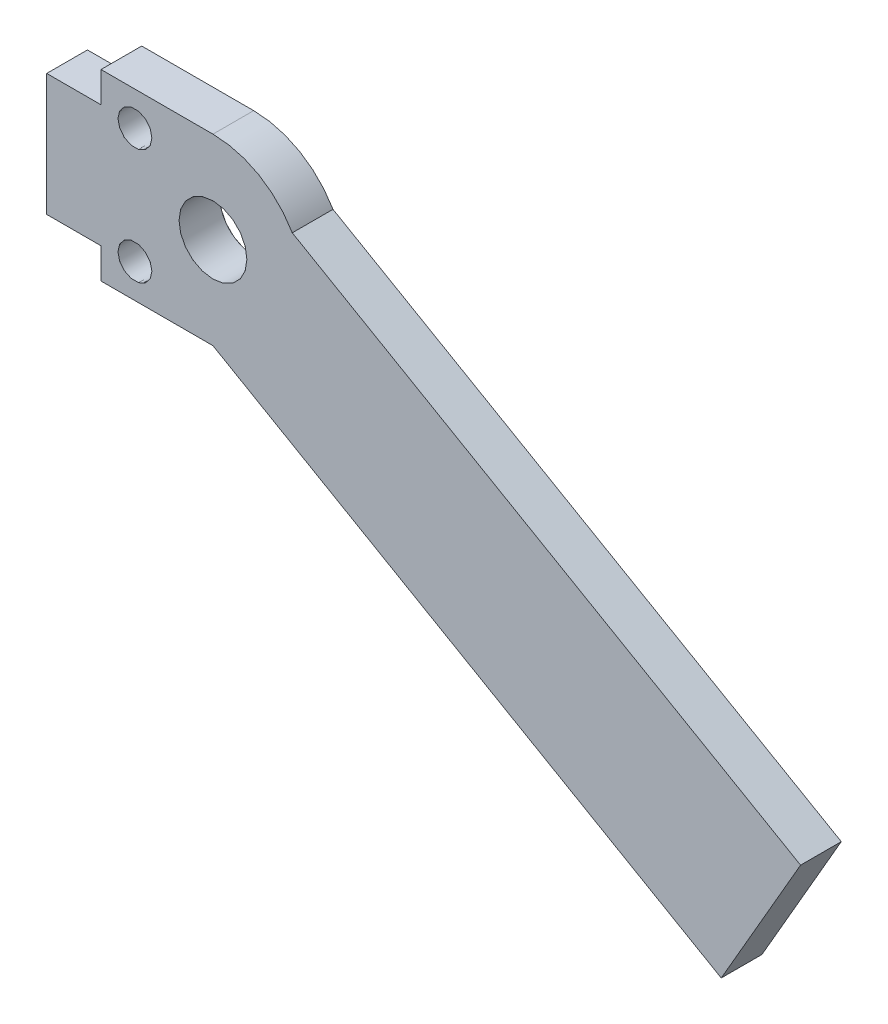
# Autodesk Inventor part: KB33-046-001-002 - Рычаг
Saved by Autodesk Inventor 2020 (Build 240168000, 168)
## iProperties
Created: 2021-06-20
Part Number: KB33-046-001-002 - Рычаг
Material: Типовые
Document SubType Name: Modeling
Designer: Петров Иван
Mass: 16.0118 g
Surface Area: 74.3338 cm^2
Volume: 16.0118 cm^3
Density: 1 g/cm^3
Appearance: По умолчанию
Author: Петров Иван
Autodesk Inventor part; units mm, degrees
ref_plane "YZ Plane" through (0, 0, 0) normal (1, 0, 0) x (0, 1, 0)
ref_plane "XZ Plane" through (0, 0, 0) normal (0, 1, 0) x (-1, 0, 0)
ref_plane "XY Plane" through (0, 0, 0) normal (0, 0, 1) x (1, 0, 0)
sketch "Эскиз1" plane through (0, 0, 0) normal (0, 0, 1) x (1, 0, 0)
  circle A0 centre (-11.5, -8.5) radius 2.5
  circle A1 centre (-11.5, 8.5) radius 2.5
  circle A2 centre (0, 0) radius 5
  arc A3 (0, -13.5) -> (0, 13.5) centre (0, 0) ccw
  line L0 (-16.5, 13.5) -> (0, 13.5)
  line L1 (-16.5, 9) -> (-16.5, 13.5)
  line L2 (-16.5, 9) -> (-24.5, 9)
  line L3 (-24.5, 9) -> (-24.5, -9)
  line L4 (-16.5, -9) -> (-24.5, -9)
  line L5 (-16.5, -13.5) -> (-16.5, -9)
  line L6 (-16.5, -13.5) -> (0, -13.5)
  point P0 (-32.5, -16)
  constraints: 14 end point, 4 centre point, 2 point on circle
extrude "Выдавливание1" add sketch "Эскиз1" along normal blind 6
sketch "Эскиз2" plane through (0, 0, 6) normal (0, 0, 1) x (1, 0, 0)
  arc A0 (0, -13.5) -> (0, 13.5) centre (0, 0) ccw projected
  line L0 (0, 13.5) -> (86.6025, -36.5)
  line L1 (86.6025, -36.5) -> (74.9112, -56.75)
  line L2 (74.9112, -56.75) -> (0, -13.5)
  line L3 (0, 13.5) -> (-16.5, 13.5) projected
  point P0 (11.6913, 6.75)
  dimension "d2" = 150
  dimension "d3" = 100
  constraints: 6 end point, 1 parallel, 1 perpendicular
  measures "d2" angle of L3 L0
  measures "d3" distance of L0.start L0.end
extrude "Выдавливание2" add sketch "Эскиз2" against normal blind 6 contours A0 L0 L1 L2
